Test diametre tube (Autodesk Fusion 360 design; units mm, degrees)
Autodesk Fusion 360 part; units mm, degrees
sketch "Sketch1" plane through (0, 0, 0) normal (0, 0, 1) x (1, 0, 0)
  circle A0 centre (0, 0) radius 5.25
  circle A1 centre (0, 0) radius 8.25
  dimension "d1" = 10.5
  dimension "d2" = 3
  constraint coincident A0.centre A1.centre
  measures "d1" diameter of A0
extrude "Extrude1" add sketch "Sketch1" along normal blind 10
sketch "Sketch2" plane through (0, 0, 10) normal (0, 0, 1) x (-1, 0, 0)
  circle A0 centre (0, 0) radius 5.25
  circle A1 centre (0, 0) radius 8.25
  circle A2 centre (0, 0) radius 5.5
  circle A3 centre (0, 0) radius 8.25
  dimension "d5" = 11
  constraint concentric A0 A2
  constraint concentric A2 A3
  measures "d5" diameter of A2
extrude "Extrude2" add sketch "Sketch2" along normal blind 10 contours A1 A3
